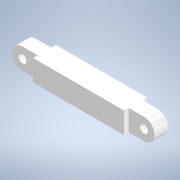
# Autodesk Inventor part: RearArm
Saved by Autodesk Inventor 2021 (Build 250183000, 183)
## iProperties
Created: 2021-05-26
Part Number: RearArm
Material: PC/ABS Plastic
Document SubType Name: Modeling
Designer: sami8
Density: 0.357273 g/cm^3
Appearance: Smooth - White
Author: sami8
Autodesk Inventor part; units mm, degrees
ref_plane "YZ Plane" through (0, 0, 0) normal (1, 0, 0) x (0, 1, 0)
ref_plane "XZ Plane" through (0, 0, 0) normal (0, 1, 0) x (-1, 0, 0)
ref_plane "XY Plane" through (0, 0, 0) normal (0, 0, 1) x (1, 0, 0)
sketch "Sketch1" plane through (0, 0, 0) normal (0, 0, 1) x (1, 0, 0)
  line L0 (-40, 0) -> (40, 0) construction
  line L1 (-40, -7) -> (40, -7)
  line L2 (40, 7) -> (-40, 7)
  arc A0 (-40, 7) -> (-40, -7) centre (-40, 0) ccw
  arc A1 (40, -7) -> (40, 7) centre (40, 0) ccw
  line L3 (-30, 7) -> (30, 7)
  line L4 (30, 7) -> (30, -7)
  line L5 (30, -7) -> (-30, -7)
  line L6 (-30, -7) -> (-30, 7)
  line L7 (-30, 7) -> (30, -7) construction
  line L8 (30, 7) -> (-30, -7) construction
  circle A2 centre (-40, 0) radius 2.6
  circle A3 centre (40, 0) radius 2.6
  circle A4 centre (0, 0) radius 1.55
  circle A5 centre (-16, 0) radius 1.55
  circle A6 centre (16, 0) radius 1.55
  dimension "d0" = 40
  dimension "d1" = 14
  dimension "d2" = 60
  dimension "d3" = 5.2
  dimension "d4" = 5.2
  dimension "d9" = 3.1
  dimension "d10" = 3.1
  dimension "d11" = 3.1
  dimension "d12" = 16
  dimension "d13" = 16
  constraints: 20 end point, 7 centre point, 4 point on circle, 4 tangent, 3 coincident, 3 midpoint, 3 parallel, 3 point on line, 2 horizontal, 1 perpendicular
  measures "d0" distance of point (0, 0) L0.end
  measures "d1" diameter of A1
  measures "d2" distance of L4.end L5.end
  measures "d3" diameter of A2
  measures "d4" diameter of A3
  measures "d9" diameter of A4
  measures "d10" diameter of A5
  measures "d11" diameter of A6
  measures "d12" distance of point (0, 0) A5.centre
  measures "d13" distance of point (0, 0) A6.centre
extrude "Extrusion1" add sketch "Sketch1" along normal mid plane 8.5
extrude "Extrusion2" add sketch "Sketch1" along normal mid plane 15 contours L6 L2 L4 L1
body "Solid1"
